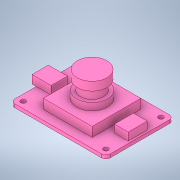
# Autodesk Inventor part: KCSU5380
Saved by Autodesk Inventor 2020 (Build 240168000, 168)
## iProperties
Created: 2018-06-08
Part Number: KCSU5380
Material: 一般
Document SubType Name: Modeling
Designer: taka
Density: 1 g/cm^3
Appearance: ピンク
Mass: 6.74398 g
Surface Area: 44.2093 cm^2
Volume: 6.74398 cm^3
Category: 頭
Author: taka
Autodesk Inventor part; units mm, degrees
ref_plane "YZ Plane" through (0, 0, 0) normal (1, 0, 0) x (0, 1, 0)
ref_plane "XZ Plane" through (0, 0, 0) normal (0, 1, 0) x (-1, 0, 0)
ref_plane "XY Plane" through (0, 0, 0) normal (0, 0, 1) x (1, 0, 0)
sketch "スケッチ1" plane through (0, 0, 0) normal (0, 1, 0) x (-1, 0, 0)
  line L0 (0, 0) -> (32, 0)
  line L1 (32, 0) -> (32, -45)
  line L2 (32, -45) -> (0, -45)
  line L3 (0, -45) -> (0, 0)
  circle A0 centre (29, -3) radius 1.15
  circle A1 centre (29, -42) radius 1.15
  circle A2 centre (3, -3) radius 1.15
  circle A3 centre (3, -42) radius 1.15
  dimension "d0" = 45
  dimension "d1" = 32
  dimension "d2" = 2.3
  dimension "d3" = 2.3
  dimension "d4" = 2.3
  dimension "d5" = 2.3
  dimension "d16" = 39
  dimension "d17" = 26
  dimension "d18" = 3
  dimension "d19" = 3
  dimension "d20" = 26
  dimension "d21" = 39
  constraints: 8 end point, 4 centre point, 2 parallel, 1 horizontal, 1 perpendicular
  measures "d0" distance between parallel lines of L2 L0
  measures "d1" distance between parallel lines of L3 L1
  measures "d2" diameter of A0
  measures "d3" diameter of A1
  measures "d4" diameter of A2
  measures "d5" diameter of A3
  measures "d16" distance of A0.centre A1.centre
  measures "d17" distance of A3.centre A1.centre
  measures "d18" distance from line of L1 A1.centre
  measures "d19" distance from line of L2 A1.centre
  measures "d20" distance of A2.centre A0.centre
  measures "d21" distance of A2.centre A3.centre
extrude "押し出し1" add sketch "スケッチ1" along normal blind 1.6
sketch "スケッチ2" plane through (0, 1.6, 0) normal (0, 1, 0) x (1, 0, 0)
  line L0 (-20.5, 37.5) -> (-11.5, 37.5)
  line L1 (-11.5, 37.5) -> (-11.5, 44)
  line L2 (-11.5, 44) -> (-20.5, 44)
  line L3 (-20.5, 44) -> (-20.5, 37.5)
  line L4 (-19.85, -2) -> (-12.15, -2)
  line L5 (-12.15, -2) -> (-12.15, 7)
  line L6 (-12.15, 7) -> (-19.85, 7)
  line L7 (-19.85, 7) -> (-19.85, -2)
  line L8 (-27.5, 11) -> (-4.5, 11)
  line L9 (-4.5, 11) -> (-4.5, 34)
  line L10 (-4.5, 34) -> (-27.5, 34)
  line L11 (-27.5, 34) -> (-27.5, 11)
  line L12 (0, 45) -> (-32, 45) projected
  line L13 (-32, 0) -> (0, 0) projected
  line L14 (-16, 0) -> (-16, 45) construction
  line L15 (-1.3785, 22.5) -> (-33.3785, 22.5) construction
  line L16 (-32, 45) -> (-32, 0) projected
  dimension "d22" = 9
  dimension "d23" = 7.7
  dimension "d25" = 23
  dimension "d26" = 23
  dimension "d27" = 9
  dimension "d28" = 6.5
  dimension "d29" = 1
  dimension "d30" = 2
  dimension "d31" = 11.5
  dimension "d32" = 11.5
  dimension "d33" = 3.85
  dimension "d34" = 4.5
  dimension "d35" = 22.5
  dimension "d36" = 45
  constraints: 28 end point, 6 parallel, 5 perpendicular, 3 horizontal, 2 midpoint
  measures "d22" distance of L2.end L1.end
  measures "d23" distance of L6.end L5.end
  measures "d25" distance of L10.end L9.end
  measures "d26" distance of L9.end L8.end
  measures "d27" distance between parallel lines of L6 L4
  measures "d28" distance between parallel lines of L2 L0
  measures "d29" distance between parallel lines of L2 L12
  measures "d30" distance between parallel lines of L4 L13
  measures "d31" distance between parallel lines of L9 L14
  measures "d32" distance between parallel lines of L15 L8
  measures "d33" distance between parallel lines of L5 L14
  measures "d34" distance between parallel lines of L1 L14
  measures "d35" distance between parallel lines of L13 L15
  measures "d36" distance of L12.end L13.start
fillet "フィレット1" radius 2 4 edges at (-32, 0.8, -45) (0, 0.8, -45) (-32, 0.8, 0) (0, 0.8, 0)
extrude "押し出し2" add sketch "スケッチ2" along normal blind 3.9 contours L7 L13 L5 L4 | L7 L6 L5 L13
sketch "スケッチ3" plane through (0, 1.6, 0) normal (0, 1, 0) x (1, 0, 0)
  line L0 (-20.5, 37.5) -> (-11.5, 37.5)
  line L1 (-11.5, 37.5) -> (-11.5, 44)
  line L2 (-11.5, 44) -> (-20.5, 44)
  line L3 (-20.5, 44) -> (-20.5, 37.5)
  line L4 (-19.85, -2) -> (-12.15, -2)
  line L5 (-12.15, -2) -> (-12.15, 7)
  line L6 (-12.15, 7) -> (-19.85, 7)
  line L7 (-19.85, 7) -> (-19.85, -2)
  line L8 (-27.5, 11) -> (-4.5, 11)
  line L9 (-4.5, 11) -> (-4.5, 34)
  line L10 (-4.5, 34) -> (-27.5, 34)
  line L11 (-27.5, 34) -> (-27.5, 11)
  line L12 (0, 45) -> (-32, 45)
  line L13 (-32, 0) -> (0, 0)
  line L14 (-16, 0) -> (-16, 45) construction
  line L15 (-1.3785, 22.5) -> (-33.3785, 22.5) construction
  line L16 (-32, 45) -> (-32, 0)
  dimension "d39" = 9
  dimension "d40" = 7.7
  dimension "d41" = 23
  dimension "d42" = 23
  dimension "d43" = 9
  dimension "d44" = 6.5
  dimension "d45" = 1
  dimension "d46" = 2
  dimension "d47" = 11.5
  dimension "d48" = 11.5
  dimension "d49" = 3.85
  dimension "d50" = 4.5
  dimension "d51" = 22.5
  dimension "d52" = 45
  constraints: 34 end point, 6 parallel, 5 perpendicular, 3 horizontal, 2 midpoint
  measures "d39" distance of L3.start L2.start
  measures "d40" distance of L7.start L5.end
  measures "d41" distance of L10.end L10.start
  measures "d42" distance of L10.start L9.start
  measures "d43" distance between parallel lines of L6 L4
  measures "d44" distance between parallel lines of L2 L0
  measures "d45" distance between parallel lines of L2 L12
  measures "d46" distance between parallel lines of L4 L13
  measures "d47" distance between parallel lines of L9 L14
  measures "d48" distance between parallel lines of L15 L8
  measures "d49" distance between parallel lines of L5 L14
  measures "d50" distance between parallel lines of L1 L14
  measures "d51" distance between parallel lines of L13 L15
  measures "d52" distance of L12.end L16.end
extrude "押し出し3" add sketch "スケッチ3" along normal blind 3.7 contours L3 L2 L1 L0
sketch "スケッチ4" plane through (0, 1.6, 0) normal (0, 1, 0) x (1, 0, 0)
  line L0 (-20.5, 37.5) -> (-11.5, 37.5)
  line L1 (-11.5, 37.5) -> (-11.5, 44)
  line L2 (-11.5, 44) -> (-20.5, 44)
  line L3 (-20.5, 44) -> (-20.5, 37.5)
  line L4 (-19.85, -2) -> (-12.15, -2)
  line L5 (-12.15, -2) -> (-12.15, 7)
  line L6 (-12.15, 7) -> (-19.85, 7)
  line L7 (-19.85, 7) -> (-19.85, -2)
  line L8 (-27.5, 11) -> (-4.5, 11)
  line L9 (-4.5, 11) -> (-4.5, 34)
  line L10 (-4.5, 34) -> (-27.5, 34)
  line L11 (-27.5, 34) -> (-27.5, 11)
  line L12 (0, 45) -> (-32, 45)
  line L13 (-32, 0) -> (0, 0)
  line L14 (-16, 0) -> (-16, 45) construction
  line L15 (-1.3785, 22.5) -> (-33.3785, 22.5) construction
  line L16 (-32, 45) -> (-32, 0)
  dimension "d55" = 9
  dimension "d56" = 7.7
  dimension "d57" = 23
  dimension "d58" = 23
  dimension "d59" = 9
  dimension "d60" = 6.5
  dimension "d61" = 1
  dimension "d62" = 2
  dimension "d63" = 11.5
  dimension "d64" = 11.5
  dimension "d65" = 3.85
  dimension "d66" = 4.5
  dimension "d67" = 22.5
  dimension "d68" = 45
  constraints: 34 end point, 6 parallel, 5 perpendicular, 3 horizontal, 2 midpoint
  measures "d55" distance of L3.start L2.start
  measures "d56" distance of L7.start L5.end
  measures "d57" distance of L10.end L10.start
  measures "d58" distance of L10.start L9.start
  measures "d59" distance between parallel lines of L6 L4
  measures "d60" distance between parallel lines of L2 L0
  measures "d61" distance between parallel lines of L2 L12
  measures "d62" distance between parallel lines of L4 L13
  measures "d63" distance between parallel lines of L9 L14
  measures "d64" distance between parallel lines of L15 L8
  measures "d65" distance between parallel lines of L5 L14
  measures "d66" distance between parallel lines of L1 L14
  measures "d67" distance between parallel lines of L13 L15
  measures "d68" distance of L12.end L16.end
extrude "押し出し4" add sketch "スケッチ4" along normal blind 4.5 contours L11 L10 L9 L8
sketch "スケッチ5" plane through (0, 6.1, 0) normal (0, 1, 0) x (1, 0, 0)
  circle A0 centre (-16, 22.5) radius 7.25
  line L0 (0, 2) -> (0, 43) projected
  point P0 (0, 0)
  dimension "d71" = 14.5
  dimension "d72" = 22.5
  dimension "d73" = 16
  constraints: 1 centre point
  measures "d71" diameter of A0
  measures "d72" vertical distance of point (0, 0) A0.centre
  measures "d73" distance from line of L0 A0.centre
extrude "押し出し5" add sketch "スケッチ5" along normal blind 3.4
sketch "スケッチ6" plane through (-16, 9.5, -22.5) normal (0, 1, 0) x (1, 0, 0)
  circle A0 centre (0, 0) radius 5.5
  circle A1 centre (0, 0) radius 7.25 projected
  point P0 (16, -22.5)
  dimension "d76" = 11
  constraints: 1 centre point, 1 concentric
  measures "d76" diameter of A0
extrude "押し出し6" add sketch "スケッチ6" along normal blind 4.5 contours A0
sketch "スケッチ7" plane through (-16, 14, -22.5) normal (0, 1, 0) x (1, 0, 0)
  circle A0 centre (0, 0) radius 7
  circle A1 centre (0, 0) radius 5.5 projected
  point P0 (16, -22.5)
  dimension "d79" = 14
  constraints: 1 centre point, 1 concentric
  measures "d79" diameter of A0
extrude "押し出し7" add sketch "スケッチ7" along normal blind 4 contours A0 | A1
equation "\"d3\" = d2"
equation "\"d4\" = d2"
equation "\"d5\" = d2"
equation "\"d20\" = d17"
equation "\"d21\" = d16"
equation "\"d31\" = 0.5 * d25"
equation "\"d32\" = 0.5 * d26"
equation "\"d33\" = 0.5 * d23"
equation "\"d34\" = 0.5 * d22"
equation "\"d35\" = 0.5 * d36"
equation "\"d47\" = 0.5 * d41"
equation "\"d48\" = 0.5 * d42"
equation "\"d49\" = 0.5 * d40"
equation "\"d50\" = 0.5 * d39"
equation "\"d51\" = 0.5 * d52"
equation "\"d63\" = 0.5 * d57"
equation "\"d64\" = 0.5 * d58"
equation "\"d65\" = 0.5 * d56"
equation "\"d66\" = 0.5 * d55"
equation "\"d67\" = 0.5 * d68"
